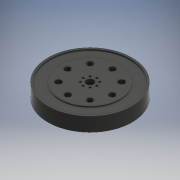
# Autodesk Inventor part: CS03
Saved by Autodesk Inventor 2017 (Build 210142000, 142)
## iProperties
Created: 2019-11-06
Part Number: CS03
Material: ABS Plastic
Document SubType Name: Modeling
Designer: Dell
Density: 1.06 g/cm^3
Appearance: Smooth - Black
Author: Dell
Autodesk Inventor part; units mm, degrees
ref_plane "YZ Plane" through (0, 0, 0) normal (1, 0, 0) x (0, 1, 0)
ref_plane "XZ Plane" through (0, 0, 0) normal (0, 1, 0) x (-1, 0, 0)
ref_plane "XY Plane" through (0, 0, 0) normal (0, 0, 1) x (1, 0, 0)
sketch "Sketch1" plane through (0, 0, 0) normal (0, 0, 1) x (1, 0, 0)
  circle A0 centre (0, 0) radius 40.5
  circle A1 centre (0, 0) radius 55.5
  dimension "d0" = 81
  dimension "d1" = 111
  constraints: 2 centre point, 2 coincident
  measures "d0" diameter of A0
  measures "d1" diameter of A1
extrude "Extrusion1" add sketch "Sketch1" along normal blind 7 contours A0 | A1
sketch "Sketch2" plane through (0, 0, 7) normal (0, 0, 1) x (1, 0, 0)
  circle A0 centre (0, 0) radius 55.5 projected
  circle A1 centre (0, 0) radius 53
  dimension "d4" = 106
  constraints: 1 centre point, 1 coincident
  measures "d4" diameter of A1
extrude "Extrusion2" add sketch "Sketch2" along normal blind 1.5
chamfer "Chamfer1" distance 1.5 angle 15 1 edges at (-53, 0, 7) measured on face at (-39.499, -35.3388, 8)
sketch "Sketch3" plane through (0, 0, 7) normal (0, 0, 1) x (1, 0, 0)
  circle A0 centre (0, 0) radius 5
  dimension "d10" = 10
  constraints: 1 centre point, 1 coincident
  measures "d10" diameter of A0
extrude "Extrusion3" cut sketch "Sketch3" against normal through all
sketch "Sketch4" plane through (0, 0, 7) normal (0, 0, 1) x (1, 0, 0)
  circle A0 centre (0, 0) radius 5 projected
  circle A1 centre (0, 0) radius 39.5
  dimension "d13" = 79
  constraints: 1 centre point, 1 coincident
  measures "d13" diameter of A1
extrude "Extrusion4" add sketch "Sketch4" along normal blind 1.5
sketch "Sketch5" plane through (0, 0, 8.5) normal (0, 0, 1) x (1, 0, 0)
  circle A0 centre (9, 0) radius 1.5
  circle A1 centre (6.364, 6.364) radius 1.5
  circle A2 centre (0, 9) radius 1.5
  circle A3 centre (-6.364, 6.364) radius 1.5
  circle A4 centre (-9, 0) radius 1.5
  circle A5 centre (-6.364, -6.364) radius 1.5
  circle A6 centre (0, -9) radius 1.5
  circle A7 centre (6.364, -6.364) radius 1.5
  point P0 (0, 0)
  dimension "d16" = 3
  dimension "d17" = 9
  dimension "d20" = 360
  constraints: 8 centre point, 1 horizontal alignment, 17 other
  measures "d16" diameter of A0
  measures "d17" distance of A0.centre point (0, 0)
extrude "Extrusion5" cut sketch "Sketch5" against normal through all
sketch "Sketch7" plane through (0, 0, 0) normal (0, 0, -1) x (-1, 0, 0)
  circle A0 centre (29.5, 0) radius 2
  circle A1 centre (20.8597, 20.8597) radius 2
  circle A2 centre (0, 29.5) radius 2
  circle A3 centre (-20.8597, 20.8597) radius 2
  circle A4 centre (-29.5, 0) radius 2
  circle A5 centre (-20.8597, -20.8597) radius 2
  circle A6 centre (0, -29.5) radius 2
  circle A7 centre (20.8597, -20.8597) radius 2
  point P0 (0, 0)
  dimension "d30" = 4
  dimension "d31" = 29.5
  dimension "d34" = 360
  constraints: 8 centre point, 1 horizontal alignment, 17 other
  measures "d30" diameter of A0
  measures "d31" distance of A0.centre point (0, 0)
extrude "Extrusion7" cut sketch "Sketch7" against normal through all
sketch "Sketch8" plane through (0, 0, 0) normal (0, 0, -1) x (-1, 0, 0)
  circle A0 centre (0, -29.5) radius 2 projected
  circle A1 centre (-29.5, 0) radius 2 projected
  circle A2 centre (0, 29.5) radius 2 projected
  circle A3 centre (29.5, 0) radius 2 projected
  circle A4 centre (20.8597, 20.8597) radius 2 projected
  circle A5 centre (-20.8597, 20.8597) radius 2 projected
  circle A6 centre (-20.8597, -20.8597) radius 2 projected
  circle A7 centre (20.8597, -20.8597) radius 2 projected
  circle A8 centre (0, -9) radius 1.5 projected
  circle A9 centre (9, 0) radius 1.5 projected
  circle A10 centre (0, 9) radius 1.5 projected
  circle A11 centre (-9, 0) radius 1.5 projected
  circle A12 centre (-6.364, 6.364) radius 1.5 projected
  circle A13 centre (6.364, 6.364) radius 1.5 projected
  circle A14 centre (6.364, -6.364) radius 1.5 projected
  circle A15 centre (-6.364, -6.364) radius 1.5 projected
  circle A16 centre (0, 0) radius 5 projected
  circle A17 centre (0, 0) radius 55.5 projected
extrude "Extrusion8" add sketch "Sketch8" along normal blind 10
sketch "Sketch9" plane through (0, 0, 8.5) normal (0, 0, 1) x (1, 0, 0)
  line L0 (-4.3301, 29.5) -> (-2.1651, 33.25)
  line L1 (-2.1651, 33.25) -> (2.1651, 33.25)
  line L2 (2.1651, 33.25) -> (4.3301, 29.5)
  line L3 (4.3301, 29.5) -> (2.1651, 25.75)
  line L4 (2.1651, 25.75) -> (-2.1651, 25.75)
  line L5 (-2.1651, 25.75) -> (-4.3301, 29.5)
  line L6 (-23.9215, 17.7978) -> (-25.0422, 21.9804)
  line L7 (-25.0422, 21.9804) -> (-21.9804, 25.0422)
  line L8 (-21.9804, 25.0422) -> (-17.7978, 23.9215)
  line L9 (-17.7978, 23.9215) -> (-16.6771, 19.7389)
  line L10 (-16.6771, 19.7389) -> (-19.7389, 16.6771)
  line L11 (-19.7389, 16.6771) -> (-23.9215, 17.7978)
  line L12 (-29.5, -4.3301) -> (-33.25, -2.1651)
  line L13 (-33.25, -2.1651) -> (-33.25, 2.1651)
  line L14 (-33.25, 2.1651) -> (-29.5, 4.3301)
  line L15 (-29.5, 4.3301) -> (-25.75, 2.1651)
  line L16 (-25.75, 2.1651) -> (-25.75, -2.1651)
  line L17 (-25.75, -2.1651) -> (-29.5, -4.3301)
  line L18 (-17.7978, -23.9215) -> (-21.9804, -25.0422)
  line L19 (-21.9804, -25.0422) -> (-25.0422, -21.9804)
  line L20 (-25.0422, -21.9804) -> (-23.9215, -17.7978)
  line L21 (-23.9215, -17.7978) -> (-19.7389, -16.6771)
  line L22 (-19.7389, -16.6771) -> (-16.6771, -19.7389)
  line L23 (-16.6771, -19.7389) -> (-17.7978, -23.9215)
  line L24 (4.3301, -29.5) -> (2.1651, -33.25)
  line L25 (2.1651, -33.25) -> (-2.1651, -33.25)
  line L26 (-2.1651, -33.25) -> (-4.3301, -29.5)
  line L27 (-4.3301, -29.5) -> (-2.1651, -25.75)
  line L28 (-2.1651, -25.75) -> (2.1651, -25.75)
  line L29 (2.1651, -25.75) -> (4.3301, -29.5)
  line L30 (23.9215, -17.7978) -> (25.0422, -21.9804)
  line L31 (25.0422, -21.9804) -> (21.9804, -25.0422)
  line L32 (21.9804, -25.0422) -> (17.7978, -23.9215)
  line L33 (17.7978, -23.9215) -> (16.6771, -19.7389)
  line L34 (16.6771, -19.7389) -> (19.7389, -16.6771)
  line L35 (19.7389, -16.6771) -> (23.9215, -17.7978)
  line L36 (29.5, 4.3301) -> (33.25, 2.1651)
  line L37 (33.25, 2.1651) -> (33.25, -2.1651)
  line L38 (33.25, -2.1651) -> (29.5, -4.3301)
  line L39 (29.5, -4.3301) -> (25.75, -2.1651)
  line L40 (25.75, -2.1651) -> (25.75, 2.1651)
  line L41 (25.75, 2.1651) -> (29.5, 4.3301)
  line L42 (17.7978, 23.9215) -> (21.9804, 25.0422)
  line L43 (21.9804, 25.0422) -> (25.0422, 21.9804)
  line L44 (25.0422, 21.9804) -> (23.9215, 17.7978)
  line L45 (23.9215, 17.7978) -> (19.7389, 16.6771)
  line L46 (19.7389, 16.6771) -> (16.6771, 19.7389)
  line L47 (16.6771, 19.7389) -> (17.7978, 23.9215)
  circle A0 centre (0, 29.5) radius 2 projected
  circle A1 centre (0, 0) radius 5 projected
  point P0 (-20.8597, 20.8597)
  point P1 (-29.5, 0)
  point P2 (-20.8597, -20.8597)
  point P3 (0, -29.5)
  point P4 (20.8597, -20.8597)
  point P5 (29.5, 0)
  point P6 (20.8597, 20.8597)
  dimension "d40" = 7.5
  dimension "d43" = 360
  constraints: 96 end point, 2 coincident, 1 horizontal, 118 other
  measures "d40" distance between parallel lines of L1 L4
extrude "Extrusion9" cut sketch "Sketch9" against normal blind 5 contours L0 L1 L2 L3 L4 L5 | L6 L7 L8 L9 L10 L11 | L12 L13 L14 L15 L16 L17 | L18 L19 L20 L21 L22 L23 | L24 L25 L26 L27 L28 L29 | L30 L31 L32 L33 L34 L35 | L36 L37 L38 L39 L40 L41 | L42 L43 L44 L45 L46 L47 | A0
body "Solid1"
